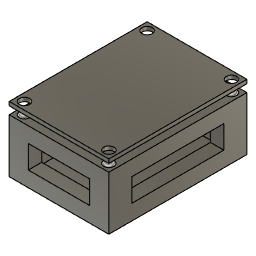
Circuit box v1 (Autodesk Fusion 360 design; units mm, degrees)
Autodesk Fusion 360 part; units mm, degrees
sketch "Sketch1" plane through (0, 0, 0) normal (0, 0, 1) x (1, 0, 0)
  line L0 (0, 0) -> (130, 0)
  line L1 (130, 0) -> (130, 180)
  line L2 (130, 180) -> (0, 180)
  line L3 (0, 180) -> (0, 0)
  dimension "d1" = 180
  dimension "d2" = 130
  constraint horizontal L0
  constraint vertical L1
  constraint horizontal L2
  constraint vertical L3
  constraint coincident L0.start L3.end
  measures "d1" distance of L0.end L1.end
  measures "d2" distance of L0.start L0.end
extrude "Extrude1" add sketch "Sketch1" along normal blind 70 makes body 1
sketch "Sketch4" plane through (0, 0, 70) normal (0, 0, 1) x (-1, 0, 0)
  line L0 (0, -180) -> (0, 0)
  line L1 (0, 0) -> (-130, 0)
  line L2 (-130, 0) -> (-130, -180)
  line L3 (-130, -180) -> (0, -180)
  line L4 (-17.5, -17.5) -> (-112.5, -17.5)
  line L5 (-112.5, -17.5) -> (-112.5, -162.5)
  line L6 (-112.5, -162.5) -> (-17.5, -162.5)
  line L7 (-17.5, -162.5) -> (-17.5, -17.5)
  line L8 (-17.5, -17.5) -> (-112.5, -162.5) construction
  line L9 (-112.5, -17.5) -> (-17.5, -162.5) construction
  point P0 (-65, -90)
  dimension "d27" = 95
  dimension "d28" = 145
  dimension "d29" = 17.5
  dimension "d30" = 17.5
  dimension "d31" = 17.5
  dimension "d32" = 17.5
  constraint horizontal L4
  constraint perpendicular L4 L5
  constraint parallel L4 L6
  constraint parallel L5 L7
  constraint coincident L8 P0
  constraint coincident L9 P0
  measures "d27" distance of L4.start L4.end
  measures "d28" distance of L4.end L5.end
  measures "d29" distance of L2 L5
  measures "d30" distance of L0 L7
  measures "d31" distance of L1 L4
  measures "d32" distance of L3 L6
extrude "Extrude4" cut sketch "Sketch4" against normal blind 60 contours L4 L5 L6 L7 bodies 1
sketch "Sketch5" plane through (0, 0, 70) normal (0, 0, 1) x (-1, 0, 0)
  line L0 (-112.5, -17.5) -> (-17.5, -17.5)
  line L1 (-17.5, -17.5) -> (-17.5, -162.5)
  line L2 (-17.5, -162.5) -> (-112.5, -162.5)
  line L3 (-112.5, -162.5) -> (-112.5, -17.5)
  line L4 (0, -180) -> (0, 0)
  line L5 (0, 0) -> (-130, 0)
  line L6 (-130, 0) -> (-130, -180)
  line L7 (-130, -180) -> (0, -180)
  circle A0 centre (-120, -10) radius 7.5
  circle A1 centre (-10, -10) radius 7.5
  circle A2 centre (-10, -170) radius 7.5
  circle A3 centre (-120, -170) radius 7.5
  dimension "d35" = 15
  dimension "d36" = 15
  dimension "d37" = 15
  dimension "d38" = 15
  dimension "d39" = 10
  dimension "d40" = 10
  dimension "d41" = 10
  dimension "d42" = 10
  dimension "d43" = 10
  dimension "d44" = 10
  dimension "d45" = 10
  dimension "d46" = 10
  measures "d35" diameter of A0
  measures "d36" diameter of A1
  measures "d37" diameter of A2
  measures "d38" diameter of A3
  measures "d39" distance of L6 A0.centre
  measures "d40" distance of L5 A0.centre
  measures "d41" distance of L5 A1.centre
  measures "d42" distance of L4 A1.centre
  measures "d43" distance of L4 A2.centre
  measures "d44" distance of L7 A2.centre
  measures "d45" distance of L6 A3.centre
  measures "d46" distance of L7 A3.centre
extrude "Extrude5" cut sketch "Sketch5" against normal blind 20 contours A0 | A1 | A2 | A3 bodies 1
thread "Thread1" "ISO Metric profile 15.0 M15x1.5 6H" major diameter 15.2033 minor diameter 13.5262 pitch 1.5 angle 60 resizes the face on face at (2.5093, 10.3738, 56.6667) on bodies 1
thread "Thread2" "ISO Metric profile 15.0 M15x1.5 6H" major diameter 15.2033 minor diameter 13.5262 pitch 1.5 angle 60 resizes the face on face at (112.5093, 10.3738, 56.6667) on bodies 1
thread "Thread3" "ISO Metric profile 15.0 M15x1.5 6H" major diameter 15.2033 minor diameter 13.5262 pitch 1.5 angle 60 resizes the face on face at (2.6487, 168.5139, 56.6667) on bodies 1
thread "Thread4" "ISO Metric profile 15.0 M15x1.5 6H" major diameter 15.2033 minor diameter 13.5262 pitch 1.5 angle 60 resizes the face on face at (127.2681, 168.1493, 56.6667) on bodies 1
sketch "Sketch6" plane through (0, 0, 0) normal (-1, 0, 0) x (0, -1, 0)
  line L0 (-180, 0) -> (0, 0)
  line L1 (0, 0) -> (0, 70)
  line L2 (0, 70) -> (-180, 70)
  line L3 (-180, 70) -> (-180, 0)
  line L4 (-30, 50) -> (-150, 50)
  line L5 (-150, 50) -> (-150, 20)
  line L6 (-150, 20) -> (-30, 20)
  line L7 (-30, 20) -> (-30, 50)
  line L8 (-30, 50) -> (-150, 20) construction
  line L9 (-150, 50) -> (-30, 20) construction
  point P0 (-90, 35)
  dimension "d57" = 120
  dimension "d58" = 30
  dimension "d59" = 90
  dimension "d60" = 35
  constraint horizontal L4
  constraint perpendicular L4 L5
  constraint parallel L4 L6
  constraint parallel L5 L7
  constraint coincident L8 P0
  constraint coincident L9 P0
  measures "d57" distance of L4.start L4.end
  measures "d58" distance of L4.start L6.end
  measures "d59" distance of L1 P0
  measures "d60" distance of L2 P0
extrude "Extrude6" cut sketch "Sketch6" against normal blind 200 contours L4 L5 L6 L7 bodies 1
sketch "Sketch7" plane through (0, 0, 0) normal (0, -1, 0) x (1, 0, 0)
  line L0 (0, 0) -> (130, 0)
  line L1 (130, 0) -> (130, 70)
  line L2 (130, 70) -> (0, 70)
  line L3 (0, 70) -> (0, 0)
  line L4 (105, 50) -> (25, 50)
  line L5 (25, 50) -> (25, 20)
  line L6 (25, 20) -> (105, 20)
  line L7 (105, 20) -> (105, 50)
  line L8 (105, 50) -> (25, 20) construction
  line L9 (25, 50) -> (105, 20) construction
  point P0 (65, 35)
  dimension "d63" = 80
  dimension "d64" = 30
  dimension "d65" = 35
  dimension "d66" = 65
  constraint horizontal L4
  constraint perpendicular L4 L5
  constraint parallel L4 L6
  constraint parallel L5 L7
  constraint coincident L8 P0
  constraint coincident L9 P0
  measures "d63" distance of L4.start L4.end
  measures "d64" distance of L4.end L5.end
  measures "d65" distance of L2 P0
  measures "d66" distance of L1 P0
extrude "Extrude7" cut sketch "Sketch7" against normal blind 230 contours L4 L5 L6 L7 bodies 1
ref_plane "WorkPlane2" through (65, 90, 80) normal (0, 0, 1) x (1, 0, 0)
sketch "Sketch8" plane through (0, 0, 80) normal (0, 0, 1) x (1, 0, 0)
  line L0 (0, 180) -> (130, 180)
  line L1 (130, 180) -> (130, 0)
  line L2 (130, 0) -> (0, 0)
  line L3 (0, 0) -> (0, 180)
  circle A0 centre (10, 170) radius 6.7631
  circle A1 centre (120, 170) radius 6.7631
  circle A2 centre (120, 10) radius 6.7631
  circle A3 centre (10, 10) radius 6.7631
  constraint horizontal L0
  constraint vertical L1
  constraint horizontal L2
  constraint vertical L3
extrude "Extrude8" add sketch "Sketch8" along normal blind 5 separate body makes body 2
shell "Shell1" [suppressed]
